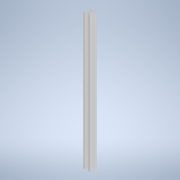
# Autodesk Inventor part: Aluminium_VSlot_1m
Saved by Autodesk Inventor 2022.2 (Build 262287000, 287)
## iProperties
Created: 2021-12-28
Part Number: Aluminium_VSlot_1m
Material: Aluminum 6061
Document SubType Name: Modeling
Designer: Radu Chirila
Density: 2.7 g/cm^3
Appearance: Aluminum - Polished
Author: Radu Chirila
Autodesk Inventor part; units mm, degrees
ref_plane "YZ Plane" through (0, 0, 0) normal (1, 0, 0) x (0, 1, 0)
ref_plane "XZ Plane" through (0, 0, 0) normal (0, 1, 0) x (-1, 0, 0)
ref_plane "XY Plane" through (0, 0, 0) normal (0, 0, 1) x (1, 0, 0)
sketch "Sketch1" plane through (0, 0, 0) normal (0, 1, 0) x (-1, 0, 0)
  line L0 (-10, 10) -> (10, 10) construction
  line L1 (10, 10) -> (10, -10) construction
  line L2 (10, -10) -> (-10, -10) construction
  line L3 (-10, -10) -> (-10, 10) construction
  line L4 (-10, 10) -> (10, -10) construction
  line L5 (10, 10) -> (-10, -10) construction
  circle A0 centre (0, 0) radius 2.1
  line L6 (-10, 0) -> (-10, -3.125) construction
  line L7 (-10, -3.125) -> (-10, 3.125) construction
  line L8 (-10, 0) -> (0, 0) construction
  line L9 (-10, 0) -> (-10, -4.7039) construction
  line L10 (-10, -4.7039) -> (-10, 4.9825) construction
  line L11 (-10, 4.9825) -> (-8.2568, 3.2393)
  line L12 (-10, -4.7039) -> (-8.2568, -2.9607)
  line L13 (-10, 0) -> (-10, -5.5) construction
  line L14 (-10, -5.5) -> (-10, 5.5) construction
  line L15 (-10, 5.5) -> (-8.2, 5.5) construction
  line L16 (-10, -5.5) -> (-8.2, -5.5) construction
  line L17 (3.9, 3.9) -> (-3.9, -3.9) construction
  line L18 (3.9, 3.9) -> (-3.9, 3.9)
  line L19 (-3.9, 3.9) -> (-3.9, -3.9)
  line L20 (-3.9, -3.9) -> (3.9, -3.9)
  line L21 (3.9, -3.9) -> (3.9, 3.9)
  line L22 (3.9, 3.9) -> (-3.9, -3.9) construction
  line L23 (-3.9, 3.9) -> (3.9, -3.9) construction
  line L24 (-8.2568, -2.9607) -> (-8.2568, -5.5)
  line L25 (-8.2568, 3.2393) -> (-8.2568, 5.5)
  line L26 (-8.2568, -5.5) -> (-6.5607, -5.5)
  line L27 (-8.2568, 5.5) -> (-6.5607, 5.5)
  line L28 (-6.5607, 5.5) -> (-3.9, 2.8393)
  line L29 (-6.5607, -5.5) -> (-3.9, -2.8393)
  line L30 (-5.5, -6.5607) -> (-2.8393, -3.9)
  line L31 (-5.5, -8.2568) -> (-5.5, -6.5607)
  line L32 (-3.2393, -8.2568) -> (-5.5, -8.2568)
  line L33 (-4.9825, -10) -> (-3.2393, -8.2568)
  line L34 (4.7039, -10) -> (2.9607, -8.2568)
  line L35 (2.9607, -8.2568) -> (5.5, -8.2568)
  line L36 (5.5, -8.2568) -> (5.5, -6.5607)
  line L37 (5.5, -6.5607) -> (2.8393, -3.9)
  line L38 (6.5607, -5.5) -> (3.9, -2.8393)
  line L39 (8.2568, -5.5) -> (6.5607, -5.5)
  line L40 (8.2568, -3.2393) -> (8.2568, -5.5)
  line L41 (10, -4.9825) -> (8.2568, -3.2393)
  line L42 (10, 4.7039) -> (8.2568, 2.9607)
  line L43 (8.2568, 2.9607) -> (8.2568, 5.5)
  line L44 (8.2568, 5.5) -> (6.5607, 5.5)
  line L45 (6.5607, 5.5) -> (3.9, 2.8393)
  line L46 (5.5, 6.5607) -> (2.8393, 3.9)
  line L47 (5.5, 8.2568) -> (5.5, 6.5607)
  line L48 (3.2393, 8.2568) -> (5.5, 8.2568)
  line L49 (4.9825, 10) -> (3.2393, 8.2568)
  line L50 (-4.7039, 10) -> (-2.9607, 8.2568)
  line L51 (-2.9607, 8.2568) -> (-5.5, 8.2568)
  line L52 (-5.5, 8.2568) -> (-5.5, 6.5607)
  line L53 (-5.5, 6.5607) -> (-2.8393, 3.9)
  line L54 (9.8, 10) -> (-9.8, 10)
  line L55 (-10, 9.8) -> (-10, -9.8)
  line L56 (-9.8, -10) -> (9.8, -10)
  line L57 (10, -9.8) -> (10, 9.8)
  line L58 (10, 10) -> (-10, -10) construction
  line L59 (-10, 10) -> (10, -10) construction
  arc A1 (-10, -9.8) -> (-9.8, -10) centre (-9.8, -9.8) ccw
  arc A2 (-9.8, 10) -> (-10, 9.8) centre (-9.8, 9.8) ccw
  arc A3 (10, 9.8) -> (9.8, 10) centre (9.8, 9.8) ccw
  arc A4 (9.8, -10) -> (10, -9.8) centre (9.8, -9.8) ccw
  line L60 (0, 3.4224) -> (0.4776, 3.9)
  line L61 (0, 3.4224) -> (-0.4776, 3.9)
  line L62 (-3.4224, 0) -> (-3.9, 0.4776)
  line L63 (-3.4224, 0) -> (-3.9, -0.4776)
  line L64 (0, -3.4224) -> (-0.4776, -3.9)
  line L65 (0, -3.4224) -> (0.4776, -3.9)
  line L66 (3.4224, 0) -> (3.9, -0.4776)
  line L67 (3.4224, 0) -> (3.9, 0.4776)
  dimension "d0" = 20
  dimension "d1" = 20
  dimension "d2" = 4.2
  dimension "d13" = 6.2
  dimension "d16" = 11
  dimension "d18" = 90
  dimension "d20" = 6.1
  dimension "d22" = 45
  dimension "d23" = 0.75
  dimension "d24" = 0.75
  dimension "d27" = 360
  dimension "d29" = 0.2
  dimension "d34" = 360
  constraints: 134 end point, 21 point on line, 8 parallel, 8 point on circle, 8 tangent, 7 midpoint, 7 perpendicular, 5 centre point, 4 horizontal, 3 equal length, 3 equal radius, 1 coincident, 1 vertical, 104 other
  measures "d0" distance of L0.end L1.end
  measures "d1" distance of L1.end L2.end
  measures "d2" diameter of A0
  measures "d13" distance of L12.end L11.end
  measures "d16" distance of L13.end L14.end
  measures "d18" angle of L12 L11
  measures "d20" distance between parallel lines of L7 L19
  measures "d22" angle to the sketch x axis of L11
  measures "d23" distance between parallel lines of L4 L28
  measures "d24" distance between parallel lines of L5 L29
  measures "d29" radius of A1
extrude "Extrusion1" add sketch "Sketch1" along normal blind 1000 contours L55 A2 L54 L50 L51 L52 L53 L18 L19 L28 L27 L25 L11 | L12 L24 L26 L29 L19 L20 L30 L31 L32 L33 L56 A1 L55 | L19 L18 L61 L60 L21 L67 L66 L20 L65 L64 L63 L62 | L54 A3 L57 L42 L43 L44 L45 L21 L18 L46 L47 L48 L49 | L34 L35 L36 L37 L20 L21 L38 L39 L40 L41 L57 A4 L56
scale "Scale1" factors (1, 0.4, 1) then translate (0, 300, 0) bodies 1
body "Solid1"
